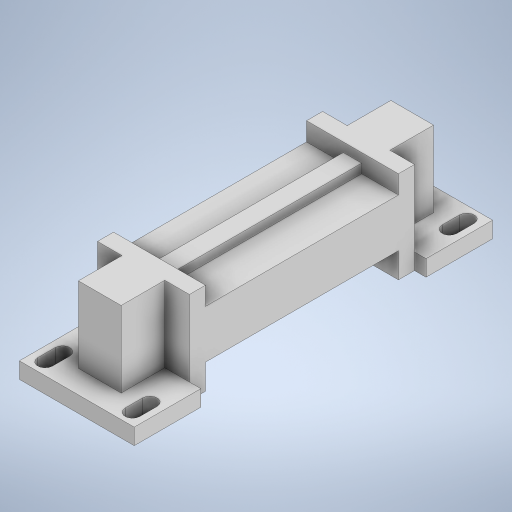
# Autodesk Inventor part: 12v_heater_mount
Saved by Autodesk Inventor 2024 (Build 280153000, 153)
## iProperties
Created: 2024-10-17
Part Number: 12v_heater_mount
Material: Generic
Document SubType Name: Modeling
Designer: Owner
Density: 1 g/cm^3
Appearance: Default
Author: Owner
Autodesk Inventor part; units mm, degrees
ref_plane "YZ Plane" through (0, 0, 0) normal (1, 0, 0) x (0, 1, 0)
ref_plane "XZ Plane" through (0, 0, 0) normal (0, 1, 0) x (-1, 0, 0)
ref_plane "XY Plane" through (0, 0, 0) normal (0, 0, 1) x (1, 0, 0)
sketch "Sketch1" plane through (0, 0, 0) normal (0, 1, 0) x (-1, 0, 0)
  line L0 (-15.875, 49.53) -> (15.875, 49.53)
  line L1 (15.875, 49.53) -> (15.875, -49.53)
  line L2 (15.875, -49.53) -> (-15.875, -49.53)
  line L3 (-15.875, -49.53) -> (-15.875, 49.53)
  line L4 (-15.875, 49.53) -> (15.875, -49.53) construction
  line L5 (15.875, 49.53) -> (-15.875, -49.53) construction
  line L6 (15.875, -49.53) -> (15.875, -48.26)
  line L7 (15.875, -49.53) -> (17.145, -49.53) construction
  line L8 (15.875, 49.53) -> (15.875, 48.26)
  line L9 (15.875, 49.53) -> (17.145, 49.53) construction
  line L10 (15.875, -49.53) -> (14.097, -49.53)
  line L11 (-15.875, -49.53) -> (-14.097, -49.53)
  line L12 (15.875, -49.53) -> (15.875, -39.37)
  line L13 (15.875, 49.53) -> (15.875, 39.37)
  line L14 (14.097, 49.53) -> (12.065, 49.53)
  line L15 (-14.097, 49.53) -> (-12.065, 49.53)
  line L16 (-12.065, -39.37) -> (-12.065, -48.26) construction
  line L17 (-10.033, -41.402) -> (-10.033, -46.228)
  line L18 (-14.097, -46.228) -> (-14.097, -41.402)
  arc A0 (-10.033, -41.402) -> (-14.097, -41.402) centre (-12.065, -41.402) ccw
  arc A1 (-14.097, -46.228) -> (-10.033, -46.228) centre (-12.065, -46.228) ccw
  line L19 (12.065, -48.26) -> (12.065, -39.37) construction
  line L20 (10.033, -46.228) -> (10.033, -41.402)
  line L21 (14.097, -41.402) -> (14.097, -46.228)
  arc A2 (10.033, -46.228) -> (14.097, -46.228) centre (12.065, -46.228) ccw
  arc A3 (14.097, -41.402) -> (10.033, -41.402) centre (12.065, -41.402) ccw
  line L22 (12.065, 39.37) -> (12.065, 48.26) construction
  line L23 (10.033, 41.402) -> (10.033, 46.228)
  line L24 (14.097, 46.228) -> (14.097, 41.402)
  arc A4 (10.033, 41.402) -> (14.097, 41.402) centre (12.065, 41.402) ccw
  arc A5 (14.097, 46.228) -> (10.033, 46.228) centre (12.065, 46.228) ccw
  line L25 (-12.065, 39.37) -> (-12.065, 48.26) construction
  line L26 (-10.033, 41.402) -> (-10.033, 46.228)
  line L27 (-14.097, 46.228) -> (-14.097, 41.402)
  arc A6 (-14.097, 41.402) -> (-10.033, 41.402) centre (-12.065, 41.402) ccw
  arc A7 (-10.033, 46.228) -> (-14.097, 46.228) centre (-12.065, 46.228) ccw
  line L28 (-12.065, 49.53) -> (-12.065, 37.6428)
  line L29 (-12.065, -37.6428) -> (-12.065, -49.53)
  line L30 (-14.097, -49.53) -> (-14.097, -39.37)
  line L31 (-14.097, 39.37) -> (-14.097, 49.53)
  line L32 (12.065, 49.53) -> (12.065, 37.6428)
  line L33 (12.065, -37.6428) -> (12.065, -49.53)
  line L34 (14.097, -49.53) -> (14.097, -39.37)
  line L35 (14.097, 39.37) -> (14.097, 49.53)
  line L36 (15.875, 39.37) -> (12.065, 39.37)
  line L37 (-12.065, 39.37) -> (-15.875, 39.37)
  line L38 (15.875, 48.26) -> (12.065, 48.26)
  line L39 (-12.065, 48.26) -> (-15.875, 48.26)
  line L40 (15.875, -39.37) -> (12.065, -39.37)
  line L41 (-12.065, -39.37) -> (-15.875, -39.37)
  line L42 (15.875, -48.26) -> (12.065, -48.26)
  line L43 (-12.065, -48.26) -> (-15.875, -48.26)
  point P0 (0, 0)
  point P1 (-12.065, -43.815)
  point P2 (12.065, -43.815)
  point P3 (12.065, 43.815)
  point P4 (-12.065, 43.815)
  dimension "d0" = 31.75
  dimension "d1" = 99.06
  dimension "d2" = 1.27
  dimension "d3" = 90
  dimension "d4" = 1.27
  dimension "d5" = 90
  dimension "d6" = 1.778
  dimension "d8" = 1.778
  dimension "d10" = 10.16
  dimension "d11" = 10.16
  dimension "d12" = 2.032
  dimension "d13" = 2.032
  constraints: 96 end point, 38 point on line, 24 point on circle, 16 tangent, 15 perpendicular, 8 centre point, 6 midpoint, 6 parallel, 3 horizontal, 2 collinear
  measures "d0" distance of L1.end L2.end
  measures "d1" distance of L0.end L1.end
  measures "d2" distance of L1.end L6.end
  measures "d3" angle of L7 L6
  measures "d4" distance of L0.end L8.end
  measures "d5" angle of L8 L9
  measures "d6" distance of L1.end L10.end
  measures "d8" distance of L2.end L11.end
  measures "d10" distance of L1.end L12.end
  measures "d11" distance of L0.end L13.end
  measures "d12" distance of L14.start L14.end
  measures "d13" distance of L15.start L15.end
extrude "Extrusion1" add sketch "Sketch1" along normal blind 4.445 contours L0 L31 L39 L3 | L0 L28 L39 L31 | L39 L31 L27 L37 L3 | L0 L32 A5 L23 A4 L36 L1 L40 A3 L20 A2 L33 L2 L29 A1 L17 A0 L41 L3 L37 A6 L26 A7 L28 | L39 A7 L31 | L0 L35 L38 L32 | L41 L30 L18 L43 L3 | L31 A6 L37 | L0 L1 L38 L35 | L38 L35 A5 | L43 L30 L2 L3 | L41 A0 L30 | L38 L1 L36 L35 L24 | A4 L35 L36 | L43 L29 L2 L30 | L30 A1 L43 | L1 L42 L34 L21 L40 | L33 L42 L34 L2 | L1 L2 L34 L42 | L34 A3 L40 | A2 L34 L42
sketch "Sketch2" plane through (0, 4.445, 0) normal (0, 1, 0) x (1, 0, 0)
  line L0 (15.875, -49.53) -> (15.875, 49.53) projected
  line L1 (-15.875, -31.115) -> (15.875, -31.115)
  line L2 (15.875, -31.115) -> (15.875, 31.115)
  line L3 (15.875, 31.115) -> (-15.875, 31.115)
  line L4 (-15.875, 31.115) -> (-15.875, -31.115)
  line L5 (-15.875, -31.115) -> (15.875, 31.115) construction
  line L6 (15.875, -31.115) -> (-15.875, 31.115) construction
  line L7 (-12.7, -31.115) -> (12.7, -31.115)
  line L8 (12.7, -31.115) -> (12.7, 31.115)
  line L9 (12.7, 31.115) -> (-12.7, 31.115)
  line L10 (-12.7, 31.115) -> (-12.7, -31.115)
  line L11 (-12.7, -31.115) -> (12.7, 31.115) construction
  line L12 (12.7, -31.115) -> (-12.7, 31.115) construction
  line L13 (-12.7, -26.67) -> (12.7, -26.67)
  line L14 (12.7, -26.67) -> (12.7, 26.67)
  line L15 (12.7, 26.67) -> (-12.7, 26.67)
  line L16 (-12.7, 26.67) -> (-12.7, -26.67)
  line L17 (-12.7, -26.67) -> (12.7, 26.67) construction
  line L18 (12.7, -26.67) -> (-12.7, 26.67) construction
  point P0 (0, 0)
  dimension "d16" = 62.23
  dimension "d19" = 25.4
  dimension "d20" = 53.34
  constraints: 36 end point, 6 midpoint, 6 parallel, 3 horizontal, 3 perpendicular, 3 point on line
  measures "d16" distance of L2.end L1.end
  measures "d19" distance of L9.end L8.end
  measures "d20" distance of L14.end L13.end
extrude "Extrusion2" cut sketch "Sketch2" against normal blind 4.445 contours L1 L8 L3 L0 | L1 L4 L3 L10 | L13 L10 L15 L8
sketch "Sketch3" plane through (0, 4.445, 0) normal (0, 1, 0) x (1, 0, 0)
  line L0 (12.7, 31.115) -> (12.7, 26.67) projected
  line L1 (-12.7, -31.115) -> (12.7, -31.115)
  line L2 (12.7, -31.115) -> (12.7, 31.115)
  line L3 (12.7, 31.115) -> (-12.7, 31.115)
  line L4 (-12.7, 31.115) -> (-12.7, -31.115)
  line L5 (-12.7, -31.115) -> (12.7, 31.115) construction
  line L6 (12.7, -31.115) -> (-12.7, 31.115) construction
  line L7 (15.875, 49.53) -> (-15.875, 49.53) projected
  line L8 (0, 49.53) -> (0, -49.53)
  line L9 (-15.875, -49.53) -> (15.875, -49.53) projected
  line L10 (0, 26.67) -> (0, 34.925)
  line L11 (12.7, -26.67) -> (-12.7, -26.67) projected
  line L12 (0, -26.67) -> (0, -34.925)
  line L13 (-12.7, 26.67) -> (12.7, 26.67) projected
  line L14 (-5.9055, 43.18) -> (5.9055, 43.18)
  line L15 (5.9055, 43.18) -> (5.9055, 26.67)
  line L16 (5.9055, 26.67) -> (-5.9055, 26.67)
  line L17 (-5.9055, 26.67) -> (-5.9055, 43.18)
  line L18 (-5.9055, 43.18) -> (5.9055, 26.67) construction
  line L19 (5.9055, 43.18) -> (-5.9055, 26.67) construction
  line L20 (-5.9055, -43.18) -> (5.9055, -43.18)
  line L21 (5.9055, -43.18) -> (5.9055, -26.67)
  line L22 (5.9055, -26.67) -> (-5.9055, -26.67)
  line L23 (-5.9055, -26.67) -> (-5.9055, -43.18)
  line L24 (-5.9055, -43.18) -> (5.9055, -26.67) construction
  line L25 (5.9055, -43.18) -> (-5.9055, -26.67) construction
  point P0 (0, 0)
  point P1 (-5.9055, -31.115)
  point P2 (5.9055, -31.115)
  point P3 (-5.9055, 31.115)
  point P4 (5.9055, 31.115)
  dimension "d23" = 8.255
  dimension "d24" = 8.255
  dimension "d25" = 11.811
  constraints: 42 end point, 9 midpoint, 6 parallel, 6 point on line, 3 horizontal, 3 perpendicular
  measures "d23" distance of L10.start L10.end
  measures "d24" distance of L12.start L12.end
  measures "d25" distance of L15.end L16.end
extrude "Extrusion3" add sketch "Sketch3" along normal blind 20.955
sketch "Sketch4" plane through (0, 25.4, 0) normal (0, 1, 0) x (1, 0, 0)
  line L0 (12.7, -26.67) -> (-12.7, -26.67) projected
  line L1 (-12.7, 26.67) -> (12.7, 26.67)
  line L2 (12.7, 26.67) -> (12.7, -26.67)
  line L3 (12.7, -26.67) -> (-12.7, -26.67)
  line L4 (-12.7, -26.67) -> (-12.7, 26.67)
  line L5 (-12.7, 26.67) -> (12.7, -26.67) construction
  line L6 (12.7, 26.67) -> (-12.7, -26.67) construction
  point P0 (0, 0)
  constraints: 12 end point, 2 midpoint, 2 parallel, 1 horizontal, 1 perpendicular
extrude "Extrusion4" cut sketch "Sketch4" against normal blind 2.54
sketch "Sketch5" plane through (0, 22.86, 0) normal (0, 1, 0) x (1, 0, 0)
  line L0 (12.7, -26.67) -> (12.7, 26.67) projected
  line L1 (-12.7, 26.67) -> (12.7, 26.67)
  line L2 (12.7, 26.67) -> (12.7, -26.67)
  line L3 (12.7, -26.67) -> (-12.7, -26.67)
  line L4 (-12.7, -26.67) -> (-12.7, 26.67)
  line L5 (-12.7, 26.67) -> (12.7, -26.67) construction
  line L6 (12.7, 26.67) -> (-12.7, -26.67) construction
  line L7 (-2.54, 26.67) -> (2.54, 26.67)
  line L8 (2.54, 26.67) -> (2.54, -26.67)
  line L9 (2.54, -26.67) -> (-2.54, -26.67)
  line L10 (-2.54, -26.67) -> (-2.54, 26.67)
  line L11 (-2.54, 26.67) -> (2.54, -26.67) construction
  line L12 (2.54, 26.67) -> (-2.54, -26.67) construction
  point P0 (0, 0)
  dimension "d28" = 5.08
  constraints: 24 end point, 4 midpoint, 4 parallel, 2 horizontal, 2 perpendicular, 1 point on line
  measures "d28" distance of L8.end L9.end
extrude "Extrusion5" cut sketch "Sketch5" against normal blind 2.54 contours L3 L8 L1 L0 | L3 L4 L1 L10
sketch "Sketch6" plane through (0, 4.445, 0) normal (0, -1, 0) x (1, 0, 0)
  line L0 (12.7, -26.67) -> (12.7, 26.67) projected
  line L1 (-12.7, 26.67) -> (12.7, 26.67)
  line L2 (12.7, 26.67) -> (12.7, -26.67)
  line L3 (12.7, -26.67) -> (-12.7, -26.67)
  line L4 (-12.7, -26.67) -> (-12.7, 26.67)
  line L5 (-12.7, 26.67) -> (12.7, -26.67) construction
  line L6 (12.7, 26.67) -> (-12.7, -26.67) construction
  line L7 (-2.54, 26.67) -> (2.54, 26.67)
  line L8 (2.54, 26.67) -> (2.54, -26.67)
  line L9 (2.54, -26.67) -> (-2.54, -26.67)
  line L10 (-2.54, -26.67) -> (-2.54, 26.67)
  line L11 (-2.54, 26.67) -> (2.54, -26.67) construction
  line L12 (2.54, 26.67) -> (-2.54, -26.67) construction
  point P0 (0, 0)
  dimension "d31" = 5.08
  constraints: 24 end point, 4 midpoint, 4 parallel, 2 horizontal, 2 perpendicular, 1 point on line
  measures "d31" distance of L8.end L9.end
extrude "Extrusion6" cut sketch "Sketch6" against normal blind 2.54 contours L3 L8 L1 L0 | L3 L4 L1 L10
equation "\"d17\" = d14"
equation "\"d14\" = 4.445"
body "Solid1"
